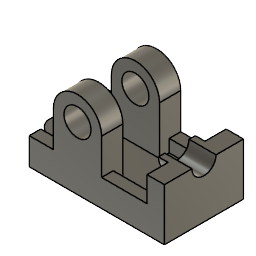
Day 6 (Autodesk Fusion 360 design; units mm, degrees)
Autodesk Fusion 360 part; units mm, degrees
note: some values were not read from the file. Set by a fixed rule: which sketch regions a step uses.
sketch "Sketch1" plane through (0, 0, 0) normal (0, 1, 0) x (1, 0, 0)
  line L0 (-100, -1.1649) -> (40, -1.1649)
  line L1 (40, -1.1649) -> (40, -55.1649)
  line L2 (40, -55.1649) -> (22, -55.1649)
  line L3 (-100, -1.1649) -> (-100, -29.1649)
  line L4 (22, -55.1649) -> (22, -29.1649)
  circle A0 centre (-50, -66.1649) radius 25
  circle A1 centre (-50, -66.1649) radius 14
  line L5 (-25, -66.1649) -> (-25, -29.1649)
  line L6 (-75, -66.1649) -> (-75, -29.1649)
  line L7 (22, -29.1649) -> (-25, -29.1649)
  line L8 (-75, -29.1649) -> (-100, -29.1649)
  line L9 (22, -29.1649) -> (40, -29.1649)
  line L10 (-100, -1.1649) -> (-117.3228, -1.1649)
  line L11 (-117.3228, -1.1649) -> (-117.3228, -16.1649)
  line L12 (-117.3228, -16.1649) -> (-100, -16.1649)
  line L13 (-100, -16.1649) -> (40, -16.1649)
  line L14 (-75, -29.1649) -> (-75, -1.1649)
  line L15 (-25, -29.1649) -> (-25, -1.1649)
  line L16 (22, -29.1649) -> (22, -1.1649)
  dimension "d1" = 140
  dimension "d2" = 54
  dimension "d3" = 18
  dimension "d6" = 28
  dimension "d7" = 50
  dimension "d8" = 28
  dimension "d9" = 65
  dimension "d10" = 90
  dimension "d11" = 15
  constraint horizontal L0
  constraint perpendicular L0 L1
  constraint perpendicular L1 L2
  constraint perpendicular L0 L3
  constraint perpendicular L2 L4
  constraint concentric A0 A1
  constraint perpendicular L3 L7
  constraint perpendicular L5 L7
  constraint coincident L6.end L7
  constraint perpendicular L6 L7
  constraint tangent A0 L6
  constraint tangent A0 L5
  constraint coincident A0 L6.start
  constraint coincident A0 L5.start
  constraint collinear L7 L8
  constraint coincident L1 L9.end
  constraint perpendicular L1 L9
  constraint perpendicular L3 L10
  constraint perpendicular L10 L11
  constraint coincident L3 L12.end
  constraint perpendicular L3 L12
  constraint coincident L1 L13.end
  constraint perpendicular L1 L13
  constraint coincident L0 L14.end
  constraint perpendicular L0 L14
  constraint coincident L0 L15.end
  constraint perpendicular L0 L15
  constraint coincident L0 L16.end
  constraint perpendicular L0 L16
  measures "d1" distance of L0.start L0.end
  measures "d2" distance of L0.end L1.end
  measures "d3" distance of L1.end L2.end
  measures "d6" distance of L0.start L3.end
  measures "d7" diameter of A0
  measures "d8" diameter of A1
  measures "d9" distance of L0 A0.centre
  measures "d10" distance of L1 A0.centre
  measures "d11" distance of L10.end L11.end
extrude "Extrude1" add sketch "Sketch1" along normal blind 82 contours L0 L3 L13 L14 | L3 L10 L11 L12 | L0 L13 L14 L15 | L0 L13 L15 L16 | L0 L1 L13 L16 | L1 L9 L13 L16 | L1 L2 L4 L9
extrude "Extrude2" add sketch "Sketch1" along normal blind 12 contours L3 L8 L13 L14 | L7 L13 L15 L16
extrude "Extrude3" add sketch "Sketch1" along normal blind 22 contours A0 L5 L6 L13 L14 L15 | A0
ref_plane "WorkPlane1" through (-38.6614, 41, 28.1649) normal (0, 1, 0) x (0, 0, 1)
mirror "Mirror1" about plane through (-38.6614, 41, 28.1649) normal (0, 1, 0) of "Extrude3"
mirror "Mirror2" about plane through (-38.6614, 41, 28.1649) normal (0, 1, 0) of "Extrude2"
sketch "Sketch2" plane through (40, 0, 0) normal (1, 0, 0) x (0, 1, 0)
  line L0 (0, 55.1649) -> (0, 1.1649)
  line L1 (0, 1.1649) -> (82, 1.1649)
  line L2 (82, 1.1649) -> (82, 55.1649)
  line L3 (82, 55.1649) -> (0, 55.1649)
  arc A0 (28.5, 55.1649) -> (53.5, 55.1649) centre (41, 55.1649) ccw
  arc A1 (21.8899, 55.1649) -> (60.1101, 55.1649) centre (41, 55.1649) ccw
  dimension "d22" = 25
  constraint midpoint L3 A0.centre
  constraint concentric A0 A1
  constraint coincident L3 A0.end
  constraint coincident L3 A0.start
  constraint coincident L3 A1.end
  constraint coincident L3 A1.start
  measures "d22" diameter of A0
extrude "Extrude4" add sketch "Sketch2" against normal blind 28 contours L3 A0 A1
extrude "Extrude5" cut sketch "Sketch2" against normal blind 28 contours L3 A0
sketch "Sketch3" plane through (0, 0, 16.1649) normal (0, 0, 1) x (-1, 0, 0)
  line L0 (-22, -70) -> (25, -70)
  line L1 (25, -70) -> (25, -60)
  line L2 (25, -60) -> (75, -60)
  line L3 (75, -60) -> (75, -70)
  line L4 (75, -70) -> (100, -70)
  line L5 (100, -70) -> (100, -82)
  line L6 (100, -82) -> (117.3228, -82)
  line L7 (117.3228, -82) -> (117.3228, 0)
  line L8 (117.3228, 0) -> (100, 0)
  line L9 (100, 0) -> (100, -12)
  line L10 (100, -12) -> (75, -12)
  line L11 (75, -12) -> (75, -22)
  line L12 (75, -22) -> (25, -22)
  line L13 (25, -22) -> (25, -12)
  line L14 (25, -12) -> (-22, -12)
  line L15 (-22, -12) -> (-22, -70)
  line L16 (100, -12) -> (100, -70) construction
  line L17 (117.3228, -41) -> (75, -41) construction
  circle A0 centre (100, -41) radius 11
  circle A1 centre (100, -41) radius 18
  line L18 (100, -12) -> (100, -70)
  dimension "d27" = 22
  dimension "d28" = 36
  constraint coincident L9.end L10.start
  constraint coincident L4.end L5.start
  constraint midpoint L7 L17.start
  constraint perpendicular L16 L17
  constraint midpoint L16 A0.centre
  constraint concentric A0 A1
  measures "d27" diameter of A0
  measures "d28" diameter of A1
extrude "Extrude6" cut sketch "Sketch3" against normal blind 30 contours L5 L6 L7 A1 L18 | L7 L8 L9 A1 L18
extrude "Extrude7" cut sketch "Sketch3" against normal blind 25 contours A0 L18 | A0 L18
equation "d28 = 18 mm + 18 mm"
